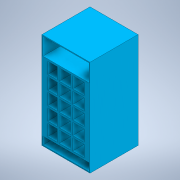
# Autodesk Inventor part: mainbox
Saved by Autodesk Inventor 2020.3 (Build 243373000, 373)
## iProperties
Created: 2021-08-07
Part Number: mainbox
Material: Stainless Steel
Document SubType Name: Modeling
Designer: 0x6f736f646f
Density: 8 g/cm^3
Appearance: Sky Blue Medium
Author: 0x6f736f646f
Autodesk Inventor part; units mm, degrees
ref_plane "YZ Plane" through (0, 0, 0) normal (1, 0, 0) x (0, 1, 0)
ref_plane "XZ Plane" through (0, 0, 0) normal (0, 1, 0) x (-1, 0, 0)
ref_plane "XY Plane" through (0, 0, 0) normal (0, 0, 1) x (1, 0, 0)
sketch "Sketch1" plane through (0, 0, 0) normal (0, 0, 1) x (1, 0, 0)
  line L0 (0, 0) -> (-500, 0)
  line L1 (-500, 1000) -> (0, 1000)
  line L2 (0, 1000) -> (0, 0)
  line L3 (-340, 530) -> (-440, 530)
  line L4 (-340, 510) -> (-440, 510)
  line L5 (-200, 530) -> (-320, 530)
  line L6 (-200, 510) -> (-320, 510)
  line L7 (-490, 810) -> (-490, 990)
  line L8 (-450, 810) -> (-490, 810)
  line L9 (-450, 790) -> (-490, 790)
  line L10 (-340, 810) -> (-440, 810)
  line L11 (-340, 790) -> (-440, 790)
  line L12 (-10, 810) -> (-50, 810)
  line L13 (-10, 790) -> (-50, 790)
  line L14 (-60, 810) -> (-180, 810)
  line L15 (-200, 810) -> (-320, 810)
  line L16 (-60, 790) -> (-180, 790)
  line L17 (-200, 790) -> (-320, 790)
  line L18 (-50, 670) -> (-50, 790)
  line L19 (-60, 670) -> (-60, 790)
  line L20 (-60, 670) -> (-180, 670)
  line L21 (-180, 530) -> (-180, 650)
  line L22 (-180, 670) -> (-180, 790)
  line L23 (-60, 650) -> (-180, 650)
  line L24 (-200, 530) -> (-200, 650)
  line L25 (-200, 670) -> (-200, 790)
  line L26 (-200, 670) -> (-320, 670)
  line L27 (-340, 530) -> (-340, 650)
  line L28 (-340, 670) -> (-340, 790)
  line L29 (-200, 650) -> (-320, 650)
  line L30 (-320, 530) -> (-320, 650)
  line L31 (-320, 670) -> (-320, 790)
  line L32 (-340, 670) -> (-440, 670)
  line L33 (-340, 650) -> (-440, 650)
  line L34 (-490, 530) -> (-490, 650)
  line L35 (-490, 670) -> (-490, 790)
  line L36 (-450, 530) -> (-450, 650)
  line L37 (-450, 670) -> (-450, 790)
  line L38 (-440, 530) -> (-440, 650)
  line L39 (-440, 670) -> (-440, 790)
  line L40 (-500, 0) -> (-500, 380)
  line L41 (-500, 390) -> (-500, 1000)
  line L42 (-450, 110) -> (-490, 110)
  line L43 (-340, 110) -> (-440, 110)
  line L44 (-200, 110) -> (-320, 110)
  line L45 (-10, 10) -> (-50, 10)
  line L46 (-450, 10) -> (-490, 10)
  line L47 (-200, 110) -> (-200, 230)
  line L48 (-180, 110) -> (-180, 230)
  line L49 (-320, 110) -> (-320, 230)
  line L50 (-200, 250) -> (-320, 250)
  line L51 (-340, 110) -> (-340, 230)
  line L52 (-200, 230) -> (-320, 230)
  line L53 (-60, 250) -> (-180, 250)
  line L54 (-60, 230) -> (-180, 230)
  line L55 (-60, 250) -> (-60, 370)
  line L56 (-50, 250) -> (-50, 370)
  line L57 (-10, 370) -> (-10, 250)
  line L58 (-180, 250) -> (-180, 370)
  line L59 (-180, 390) -> (-180, 510)
  line L60 (-200, 250) -> (-200, 370)
  line L61 (-200, 390) -> (-200, 510)
  line L62 (-60, 390) -> (-180, 390)
  line L63 (-60, 370) -> (-180, 370)
  line L64 (-320, 250) -> (-320, 370)
  line L65 (-320, 390) -> (-320, 510)
  line L66 (-200, 390) -> (-320, 390)
  line L67 (-340, 250) -> (-340, 370)
  line L68 (-340, 390) -> (-340, 510)
  line L69 (-200, 370) -> (-320, 370)
  line L70 (-340, 390) -> (-440, 390)
  line L71 (-340, 370) -> (-440, 370)
  line L72 (-450, 390) -> (-450, 510)
  line L73 (-440, 390) -> (-440, 510)
  line L74 (-490, 390) -> (-490, 510)
  line L75 (-50, 990) -> (-10, 990)
  line L76 (-180, 990) -> (-60, 990)
  line L77 (-320, 990) -> (-200, 990)
  line L78 (-490, 990) -> (-450, 990)
  line L79 (-440, 990) -> (-340, 990)
  line L80 (-340, 250) -> (-440, 250)
  line L81 (-340, 230) -> (-440, 230)
  line L82 (-450, 110) -> (-450, 230)
  line L83 (-450, 250) -> (-450, 370)
  line L84 (-440, 110) -> (-440, 230)
  line L85 (-440, 250) -> (-440, 370)
  line L86 (-490, 110) -> (-490, 230)
  line L87 (-490, 250) -> (-490, 370)
  line L88 (-10, 110) -> (-50, 110)
  line L89 (-60, 110) -> (-180, 110)
  line L90 (-60, 110) -> (-60, 230)
  line L91 (-50, 110) -> (-50, 230)
  line L92 (-10, 230) -> (-10, 110)
  line L93 (-10, 990) -> (-10, 810)
  line L94 (-10, 790) -> (-10, 670)
  line L95 (-450, 990) -> (-440, 990)
  line L96 (-340, 990) -> (-320, 990)
  line L97 (-200, 990) -> (-180, 990)
  line L98 (-60, 990) -> (-50, 990)
  line L99 (-50, 810) -> (-60, 810)
  line L100 (-180, 810) -> (-200, 810)
  line L101 (-320, 810) -> (-340, 810)
  line L102 (-440, 810) -> (-450, 810)
  line L103 (-500, 380) -> (-500, 390)
  line L104 (-60, 530) -> (-180, 530)
  line L105 (-60, 390) -> (-60, 510)
  line L106 (-60, 530) -> (-60, 650)
  line L107 (-60, 510) -> (-180, 510)
  line L108 (-50, 390) -> (-50, 510)
  line L109 (-50, 530) -> (-50, 650)
  line L110 (-10, 650) -> (-10, 530)
  line L111 (-10, 510) -> (-10, 390)
  line L112 (-10, 10) -> (-490, 10)
  line L113 (-490, 10) -> (-490, 90)
  line L114 (-490, 90) -> (-10, 90)
  line L115 (-10, 90) -> (-10, 10)
  line L116 (-450, 110) -> (-490, 110)
  line L117 (-490, 110) -> (-490, 790)
  line L118 (-490, 790) -> (-450, 790)
  line L119 (-450, 790) -> (-450, 110)
  line L120 (-50, 790) -> (-10, 790)
  line L121 (-10, 790) -> (-10, 110)
  line L122 (-10, 110) -> (-50, 110)
  line L123 (-50, 110) -> (-50, 790)
  dimension "d0" = 500
  dimension "d1" = 1000
  dimension "d32" = 10
  dimension "d33" = 40
  dimension "d34" = 10
  dimension "d35" = 100
  dimension "d36" = 10
  dimension "d37" = 50
  dimension "d38" = 10
  dimension "d39" = 120
  dimension "d40" = 20
  dimension "d41" = 120
  dimension "d42" = 120
  dimension "d43" = 10
  dimension "d44" = 80
  dimension "d45" = 480
  dimension "d46" = 10
  dimension "d47" = 10
  constraints: 248 end point, 105 parallel, 35 equal length, 23 perpendicular, 7 collinear, 5 horizontal
  measures "d0" distance of L1.start L1.end
  measures "d1" distance of L0.end L1.start
  measures "d32" distance between parallel lines of L35 L41
  measures "d33" distance between parallel lines of L37 L35
  measures "d34" distance between parallel lines of L39 L37
  measures "d35" distance between parallel lines of L39 L28
  measures "d36" distance between parallel lines of L2 L94
  measures "d37" distance between parallel lines of L2 L18
  measures "d38" distance between parallel lines of L18 L19
  measures "d39" distance between parallel lines of L19 L22
  measures "d40" distance between parallel lines of L22 L25
  measures "d41" distance between parallel lines of L25 L31
  measures "d42" distance between parallel lines of L26 L17
  measures "d43" distance between parallel lines of L110 L2
  measures "d44" distance of L112.end L113.end
  measures "d45" distance between parallel lines of L115 L113
  measures "d46" distance between parallel lines of L2 L115
  measures "d47" distance between parallel lines of L0 L112
extrude "Extrusion1" add sketch "Sketch1" along normal blind 500 contours L0 L40 L103 L41 L1 L2 | L37 L119 L36 L72 L83 L82 L42 L86 L117 L87 L74 L34 L35 L9 | L94 L121 L110 L111 L57 L92 L88 L91 L123 L56 L108 L109 L18 L13
extrude "Extrusion2" add sketch "Sketch1" along normal blind 50 contours L0 L40 L103 L41 L1 L2 | L3 L38 L33 L27 | L68 L70 L73 L4 | L5 L30 L29 L24 | L61 L66 L65 L6 | L7 L78 L95 L79 L96 L77 L97 L76 L98 L75 L93 L12 L99 L14 L100 L15 L101 L10 L102 L8 | L37 L119 L36 L72 L83 L82 L42 L86 L117 L87 L74 L34 L35 L9 | L28 L32 L39 L11 | L94 L121 L110 L111 L57 L92 L88 L91 L123 L56 L108 L109 L18 L13 | L19 L20 L22 L16 | L25 L26 L31 L17 | L21 L23 L106 L104 | L43 L84 L81 L51 | L44 L49 L52 L47 | L45 L112 L46 L113 L114 L115 | L48 L54 L90 L89 | L50 L64 L69 L60 | L53 L58 L63 L55 | L59 L107 L105 L62 | L80 L85 L71 L67
body "Solid1"
